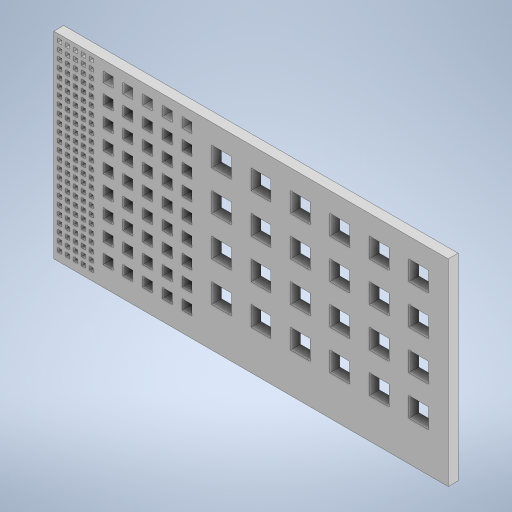
# Autodesk Inventor part: gratingdimtest
Saved by Autodesk Inventor 2023 (Build 270158000, 158)
## iProperties
Created: 2022-05-25
Part Number: gratingdimtest
Material: Generisch
Document SubType Name: Modeling
Designer: Tim Stechel
Density: 1 g/cm^3
Appearance: Vorgabe
Author: Tim Stechel
Autodesk Inventor part; units mm, degrees
ref_plane "YZ Plane" through (0, 0, 0) normal (1, 0, 0) x (0, 1, 0)
ref_plane "XZ Plane" through (0, 0, 0) normal (0, 1, 0) x (-1, 0, 0)
ref_plane "XY Plane" through (0, 0, 0) normal (0, 0, 1) x (1, 0, 0)
sketch "Skizze1" plane through (0, 0, 0) normal (0, 0, 1) x (1, 0, 0)
  line L0 (0, 0) -> (10, 0)
  line L1 (10, 0) -> (10, -10)
  line L2 (10, -10) -> (0, -10)
  line L3 (0, -10) -> (0, 0)
  line L4 (-21.1143, -5) -> (18.872, -5)
  line L5 (5, 8.9424) -> (5, -5.0722)
  line L6 (0, 0) -> (0.1, 0)
  line L7 (0.1, 0) -> (0.1, -10)
  line L8 (0.1, -10) -> (0, -10)
  line L9 (0, -10) -> (0, 0)
  line L10 (0.2, 0) -> (0.2, -10)
  line L11 (0.3, 0) -> (0.3, -10)
  line L12 (0.4, 0) -> (0.4, -10)
  line L13 (0.5, 0) -> (0.5, -10)
  line L14 (0.6, 0) -> (0.6, -10)
  line L15 (0.7, 0) -> (0.7, -10)
  line L16 (0.8, 0) -> (0.8, -10)
  line L17 (0.9, 0) -> (0.9, -10)
  line L18 (1, 0) -> (1, -10)
  line L19 (1, 0) -> (1.25, 0)
  line L20 (1.25, 0) -> (1.25, -10)
  line L21 (1.25, -10) -> (1, -10)
  line L22 (1, -10) -> (1, 0)
  line L23 (1.5, 0) -> (1.5, -10)
  line L24 (1.75, 0) -> (1.75, -10)
  line L25 (2, 0) -> (2, -10)
  line L26 (2.25, 0) -> (2.25, -10)
  line L27 (2.5, 0) -> (2.5, -10)
  line L28 (2.75, 0) -> (2.75, -10)
  line L29 (3, 0) -> (3, -10)
  line L30 (3.25, 0) -> (3.25, -10)
  line L31 (3.5, 0) -> (3.5, -10)
  line L32 (3.5, 0) -> (4, 0)
  line L33 (4, 0) -> (4, -10)
  line L34 (4, -10) -> (3.5, -10)
  line L35 (3.5, -10) -> (3.5, 0)
  line L36 (4.5, 0) -> (4.5, -10)
  line L37 (5, 0) -> (5, -10)
  line L38 (5.5, 0) -> (5.5, -10)
  line L39 (6, 0) -> (6, -10)
  line L40 (6.5, 0) -> (6.5, -10)
  line L41 (7, 0) -> (7, -10)
  line L42 (7.5, 0) -> (7.5, -10)
  line L43 (8, 0) -> (8, -10)
  line L44 (8.5, 0) -> (8.5, -10)
  line L45 (9, 0) -> (9, -10)
  line L46 (9.5, 0) -> (9.5, -10)
  point P0 (0, 0)
  point P1 (9.5, -5)
  point P2 (10, -5)
  point P3 (9, -5)
  point P4 (8.5, -5)
  point P5 (8, -5)
  point P6 (7.5, -5)
  point P7 (7, -5)
  point P8 (6.5, -5)
  point P9 (6, -5)
  point P10 (5.5, -5)
  point P11 (4.5, -5)
  point P12 (5, -5)
  point P13 (5, 0)
  point P14 (4, -5)
  point P15 (3.5, -5)
  point P16 (3.25, -5)
  point P17 (3, -5)
  point P18 (2.75, -5)
  point P19 (2.5, -5)
  point P20 (2.25, -5)
  point P21 (2, -5)
  point P22 (1.75, -5)
  point P23 (1.5, -5)
  point P24 (1.25, -5)
  point P25 (1, -5)
  point P26 (0.9, -5)
  point P27 (0.8, -5)
  point P28 (0.7, -5)
  point P29 (0.6, -5)
  point P30 (0.5, -5)
  point P31 (0.4, -5)
  point P32 (0.3, -5)
  point P33 (0.2, -5)
  point P34 (0.1, -5)
  point P35 (0, -5)
  dimension "d0" = 10
  dimension "d1" = 10
  dimension "d3" = 0.1
  dimension "d6" = 0.1
  dimension "d11" = 0.25
  dimension "d14" = 0.25
  dimension "d19" = 0.5
  dimension "d22" = 0.5
  constraints: 90 end point, 58 horizontal alignment, 36 parallel, 5 horizontal, 3 perpendicular, 3 point on line, 2 vertical, 7 other
  measures "d0" distance of L3.end L1.start
  measures "d1" distance of L1.start L1.end
  measures "d3" distance of L7.end L8.end
  measures "d6" distance of L6.end L10.start
  measures "d11" distance of L20.end L21.end
  measures "d14" distance of L19.end L23.start
  measures "d19" distance of L33.end L34.end
  measures "d22" distance of L32.end L36.start
extrude "Extrusion1" add sketch "Skizze1" along normal blind 0.25 contours L0 L7 L4 L3 | L0 L11 L4 L10 | L0 L13 L4 L12 | L0 L15 L4 L14 | L0 L17 L4 L16 | L0 L20 L4 L18 | L0 L24 L4 L23 | L0 L26 L4 L25 | L0 L28 L4 L27 | L0 L30 L4 L29 | L0 L33 L4 L31 | L0 L5 L4 L36 | L0 L39 L4 L38 | L0 L41 L4 L40 | L0 L43 L4 L42 | L0 L45 L4 L44 | L0 L1 L4 L46
sketch "Skizze2" plane through (0, 0, 0.25) normal (0, 0, 1) x (1, 0, 0)
  line L0 (0.1, 0) -> (0, 0) projected
  line L1 (1.25, -5) -> (1.25, 0) projected
  line L2 (0, 0) -> (1.25, 0)
  line L3 (1.25, 0) -> (1.25, -0.1)
  line L4 (1.25, -0.1) -> (0, -0.1)
  line L5 (0, -0.1) -> (0, 0)
  line L6 (1.25, -0.2) -> (0, -0.2)
  line L7 (1.25, -0.3) -> (0, -0.3)
  line L8 (1.25, -0.4) -> (0, -0.4)
  line L9 (1.25, -0.5) -> (0, -0.5)
  line L10 (1.25, -0.6) -> (0, -0.6)
  line L11 (1.25, -0.7) -> (0, -0.7)
  line L12 (1.25, -0.8) -> (0, -0.8)
  line L13 (1.25, -0.9) -> (0, -0.9)
  line L14 (1.25, -1) -> (0, -1)
  line L15 (1.25, -1.1) -> (0, -1.1)
  line L16 (1.25, -1.2) -> (0, -1.2)
  line L17 (1.25, -1.3) -> (0, -1.3)
  line L18 (1.25, -1.4) -> (0, -1.4)
  line L19 (1.25, -1.5) -> (0, -1.5)
  line L20 (1.25, -1.6) -> (0, -1.6)
  line L21 (1.25, -1.7) -> (0, -1.7)
  line L22 (1.25, -1.8) -> (0, -1.8)
  line L23 (1.25, -1.9) -> (0, -1.9)
  line L24 (1.25, -2) -> (0, -2)
  line L25 (1.25, -2.1) -> (0, -2.1)
  line L26 (1.25, -2.2) -> (0, -2.2)
  line L27 (1.25, -2.3) -> (0, -2.3)
  line L28 (1.25, -2.4) -> (0, -2.4)
  line L29 (1.25, -2.5) -> (0, -2.5)
  line L30 (1.25, -2.6) -> (0, -2.6)
  line L31 (1.25, -2.7) -> (0, -2.7)
  line L32 (1.25, -2.8) -> (0, -2.8)
  line L33 (1.25, -2.9) -> (0, -2.9)
  line L34 (1.25, -3) -> (0, -3)
  line L35 (1.25, -3.1) -> (0, -3.1)
  line L36 (1.25, -3.2) -> (0, -3.2)
  line L37 (1.25, -3.3) -> (0, -3.3)
  line L38 (1.25, -3.4) -> (0, -3.4)
  line L39 (1.25, -3.5) -> (0, -3.5)
  line L40 (1.25, -3.6) -> (0, -3.6)
  line L41 (1.25, -3.7) -> (0, -3.7)
  line L42 (1.25, -3.8) -> (0, -3.8)
  line L43 (1.25, -3.9) -> (0, -3.9)
  line L44 (1.25, -4) -> (0, -4)
  line L45 (1.25, -4.1) -> (0, -4.1)
  line L46 (1.25, -4.2) -> (0, -4.2)
  line L47 (1.25, -4.3) -> (0, -4.3)
  line L48 (1.25, -4.4) -> (0, -4.4)
  line L49 (1.25, -4.5) -> (0, -4.5)
  line L50 (1.25, -4.6) -> (0, -4.6)
  line L51 (1.25, -4.7) -> (0, -4.7)
  line L52 (1.25, -4.8) -> (0, -4.8)
  line L53 (1.25, -4.9) -> (0, -4.9)
  line L54 (1.25, -5) -> (0, -5)
  line L55 (0, 0) -> (1.25, 0)
  line L56 (1.25, 0) -> (1.25, -5)
  line L57 (1.25, -5) -> (0, -5)
  line L58 (0, -5) -> (0, 0)
  point P0 (0, 0)
  point P1 (0, -4.8)
  point P2 (0, -4.6)
  point P3 (0, -4.7)
  point P4 (0, -4.4)
  point P5 (0, -4.5)
  point P6 (0, -4.2)
  point P7 (0, -4.3)
  point P8 (0, -4)
  point P9 (0, -4.1)
  point P10 (0, -3.8)
  point P11 (0, -3.9)
  point P12 (0, -3.6)
  point P13 (0, -3.7)
  point P14 (0, -3.4)
  point P15 (0, -3.5)
  point P16 (0, -3.2)
  point P17 (0, -3.3)
  point P18 (0, -3)
  point P19 (0, -3.1)
  point P20 (0, -2.8)
  point P21 (0, -2.9)
  point P22 (0, -2.6)
  point P23 (0, -2.7)
  point P24 (0, -2.4)
  point P25 (0, -2.5)
  point P26 (0, -2.2)
  point P27 (0, -2.3)
  point P28 (0, -2)
  point P29 (0, -2.1)
  point P30 (0, -1.8)
  point P31 (0, -1.9)
  point P32 (0, -1.6)
  point P33 (0, -1.7)
  point P34 (0, -1.4)
  point P35 (0, -1.5)
  point P36 (0, -1.2)
  point P37 (0, -1.3)
  point P38 (0, -1)
  point P39 (0, -1.1)
  point P40 (0, -0.8)
  point P41 (0, -0.9)
  point P42 (0, -0.6)
  point P43 (0, -0.7)
  point P44 (0, -0.4)
  point P45 (0, -0.5)
  point P46 (0, -0.2)
  point P47 (0, -0.3)
  dimension "d29" = 0.1
  dimension "d32" = 0.1
  constraints: 112 end point, 3 parallel, 2 horizontal, 2 perpendicular, 2 vertical, 152 other
  measures "d29" distance of L4.end L0.end
  measures "d32" distance of L3.end L6.start
extrude "Extrusion2" add sketch "Skizze2" against normal up to surface (0.25 mm away) contours L2 L1 L4 L5 L0 | L6 L1 L7 L58 | L8 L1 L9 L58 | L10 L1 L11 L58 | L12 L1 L13 L58 | L14 L1 L15 L58 | L16 L1 L17 L58 | L18 L1 L19 L58 | L20 L1 L21 L58 | L22 L1 L23 L58 | L24 L1 L25 L58 | L26 L1 L27 L58 | L28 L1 L29 L58 | L30 L1 L31 L58 | L32 L1 L33 L58 | L34 L1 L35 L58 | L36 L1 L37 L58 | L38 L1 L39 L58 | L40 L1 L41 L58 | L42 L1 L43 L58 | L44 L1 L45 L58 | L46 L1 L47 L58 | L48 L1 L49 L58 | L50 L1 L51 L58 | L52 L1 L53 L58 | L53 L1 L54 L58
sketch "Skizze3" plane through (0, 0, 0.25) normal (0, 0, 1) x (1, 0, 0)
  line L0 (1.25, 0) -> (0, 0) projected
  line L1 (1.25, 0) -> (4, 0)
  line L2 (4, 0) -> (4, -5)
  line L3 (4, -5) -> (1.25, -5)
  line L4 (1.25, -5) -> (1.25, 0)
  line L5 (4, -5) -> (4, 0) projected
  line L6 (1.25, 0) -> (4, 0)
  line L7 (4, 0) -> (4, -0.2555)
  line L8 (1.25, -0.25) -> (1.25, 0)
  line L9 (4, 0) -> (3.5, 0) projected
  line L10 (4, 0) -> (4, -0.25)
  line L11 (4, -0.25) -> (1.25, -0.25)
  line L12 (1.25, -5) -> (1.25, 0) projected
  line L13 (1.25, 0) -> (1.25, -0.25)
  line L14 (4, -0.5) -> (1.25, -0.5)
  line L15 (4, -0.75) -> (1.25, -0.75)
  line L16 (4, -1) -> (1.25, -1)
  line L17 (4, -1.25) -> (1.25, -1.25)
  line L18 (4, -1.5) -> (1.25, -1.5)
  line L19 (4, -1.75) -> (1.25, -1.75)
  line L20 (4, -2) -> (1.25, -2)
  line L21 (4, -2.25) -> (1.25, -2.25)
  line L22 (4, -2.5) -> (1.25, -2.5)
  line L23 (4, -2.75) -> (1.25, -2.75)
  line L24 (4, -3) -> (1.25, -3)
  line L25 (4, -3.25) -> (1.25, -3.25)
  line L26 (4, -3.5) -> (1.25, -3.5)
  line L27 (4, -3.75) -> (1.25, -3.75)
  line L28 (4, -4) -> (1.25, -4)
  line L29 (4, -4.25) -> (1.25, -4.25)
  line L30 (4, -4.5) -> (1.25, -4.5)
  line L31 (4, -4.75) -> (1.25, -4.75)
  line L32 (4, -5) -> (1.25, -5)
  point P0 (0, 0)
  dimension "d39" = 0.25
  dimension "d42" = 0.25
  constraints: 58 end point, 3 parallel, 3 perpendicular, 2 horizontal, 2 point on line, 1 collinear, 1 vertical, 57 other
  measures "d39" distance of L1.end L10.end
  measures "d42" distance of L10.end L14.start
extrude "Extrusion3" add sketch "Skizze3" against normal up to surface (0.25 mm away) contours L1 L2 L11 L4 | L14 L2 L15 L4 | L16 L2 L17 L4 | L18 L2 L19 L4 | L20 L2 L21 L4 | L22 L2 L23 L4 | L24 L2 L25 L4 | L26 L2 L27 L4 | L28 L2 L29 L4 | L30 L2 L31 L4 | L31 L2 L3 L4
sketch "Skizze4" plane through (0, 0, 0.25) normal (0, 0, 1) x (1, 0, 0)
  line L0 (4, -5) -> (4, 0) projected
  line L1 (9.5, -5) -> (10, -5) projected
  line L2 (4, 0) -> (10, 0)
  line L3 (10, 0) -> (10, -5)
  line L4 (10, -5) -> (4, -5)
  line L5 (4, -5) -> (4, 0)
  line L6 (4, 0) -> (4, -0.5)
  line L7 (4, -0.5) -> (10, -0.5)
  line L8 (10, -5) -> (10, 0) projected
  line L9 (10, 0) -> (10, -0.5)
  line L10 (4, -1) -> (10, -1)
  line L11 (4, -1.5) -> (10, -1.5)
  line L12 (4, -2) -> (10, -2)
  line L13 (4, -2.5) -> (10, -2.5)
  line L14 (4, -3) -> (10, -3)
  line L15 (4, -3.5) -> (10, -3.5)
  line L16 (4, -4) -> (10, -4)
  line L17 (4, -4.5) -> (10, -4.5)
  line L18 (4, -5) -> (10, -5)
  point P0 (0, 0)
  dimension "d49" = 0.5
  dimension "d52" = 0.5
  constraints: 32 end point, 2 parallel, 2 perpendicular, 2 point on line, 1 collinear, 1 horizontal, 1 vertical, 27 other
  measures "d49" distance of L0.end L6.end
  measures "d52" distance of L6.end L10.start
extrude "Extrusion4" add sketch "Skizze4" against normal up to surface (0.25 mm away) contours L0 L17 L3 L1 L4 | L0 L16 L3 L17 | L0 L14 L3 L15 | L0 L12 L3 L13 | L0 L10 L3 L11 | L0 L2 L3 L7
